rpitouchsupportextender (Autodesk Fusion 360 design; units mm, degrees)
Autodesk Fusion 360 part; units mm, degrees
sketch "Sketch1" plane through (0, 0, 0) normal (0, 0, 1) x (1, 0, 0)
  line L0 (4.8, -5) -> (-4.8, -5)
  line L1 (-4.8, -5) -> (-4.8, 5)
  line L2 (4.8, 5) -> (4.8, -5)
  line L3 (4.8, -5) -> (-4.8, 5) construction
  line L4 (-4.8, -5) -> (4.8, 5) construction
  line L5 (-4.8, -5) -> (4.8, -5)
  line L6 (4.8, -7.5) -> (4.8, -45)
  line L7 (4.8, -45) -> (-4.8, -45)
  line L8 (-4.8, -45) -> (-4.8, -7.5)
  line L9 (-10.3, -7.5) -> (-10.3, 7.5)
  line L10 (10.3, 7.5) -> (10.3, -7.5)
  line L11 (10.3, -7.5) -> (-10.3, 7.5) construction
  line L12 (-10.3, -7.5) -> (10.3, 7.5) construction
  line L13 (4.8, 5) -> (10.3, 5)
  line L14 (-4.8, 5) -> (-10.3, 5)
  line L15 (10.3, -7.5) -> (4.8, -7.5)
  line L16 (-4.8, -7.5) -> (-10.3, -7.5)
  dimension "d1" = 9.6
  dimension "d3" = 9.6
  dimension "d4" = 40
  dimension "d5" = 20.6
  constraint horizontal L0
  constraint perpendicular L0 L1
  constraint parallel L1 L2
  constraint coincident L3 origin
  constraint coincident L4 origin
  constraint horizontal L5
  constraint vertical L6
  constraint horizontal L7
  constraint vertical L8
  constraint horizontal L15
  constraint perpendicular L9 L15
  constraint parallel L9 L10
  constraint coincident L11 origin
  constraint coincident L12 origin
  constraint coincident L10 L13.end
  constraint perpendicular L10 L13
  constraint coincident L9 L14.end
  constraint perpendicular L9 L14
  constraint collinear L15 L16
  measures "d1" distance of L1.end L2.start
  measures "d3" distance of L0.end L0.start
  measures "d4" distance of L0.end L7.end
  measures "d5" distance of L9.end L10.start
extrude "Extrude1" add sketch "Sketch1" along normal blind 10
fillet "Fillet1" radius 3.5 2 edges at (0, -45, 10) (0, -45, 0)
chamfer "Chamfer1" distance 4 angle 45 2 edges at (-4.8, -7.5, 5) (4.8, -7.5, 5)
fillet "Fillet2" radius 4.5 2 edges at (10.3, 5, 5) (-10.3, 5, 5)
